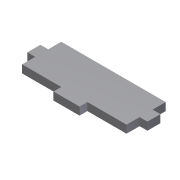
# Autodesk Inventor part: OpenROV_Dev_EChassis_Seperator
Saved by Autodesk Inventor 2012 (Build 160160000, 160)
## iProperties
Created: 2012-08-08
Part Number: OpenROV_Dev_EChassis_Seperator
Material: Default
Document SubType Name: Modeling
Designer: user
Density: 1 g/cm^3
Author: user
Autodesk Inventor part; units mm, degrees
ref_plane "YZ Plane" through (0, 0, 0) normal (1, 0, 0) x (0, 1, 0)
ref_plane "XZ Plane" through (0, 0, 0) normal (0, 1, 0) x (-1, 0, 0)
ref_plane "XY Plane" through (0, 0, 0) normal (0, 0, 1) x (1, 0, 0)
sketch "Sketch1" plane through (0, 0, 0) normal (0, 0, 1) x (1, 0, 0)
  line L0 (0, 0) -> (0, 5)
  line L1 (0, 5) -> (-3, 5)
  line L2 (-3, 5) -> (-3, 10)
  line L3 (0, 15) -> (40, 15)
  line L4 (43, 10) -> (43, 5)
  line L5 (43, 5) -> (40, 5)
  line L6 (40, 5) -> (40, 0)
  line L7 (40, 0) -> (25, 0)
  line L8 (25, 0) -> (25, -3)
  line L9 (25, -3) -> (15, -3)
  line L10 (15, -3) -> (15, 0)
  line L11 (15, 0) -> (0, 0)
  line L12 (40, 15) -> (40, 10)
  line L13 (40, 10) -> (43, 10)
  line L14 (-3, 10) -> (0, 10)
  line L15 (0, 10) -> (0, 15)
  dimension "d3" = 3
  dimension "d5" = 15
  dimension "d6" = 3
  dimension "d7" = 10
  dimension "d8" = 3
  dimension "d9" = 15
  dimension "d14" = 5
  dimension "d15" = 15
  dimension "d16" = 5
  dimension "d17" = 5
  dimension "d18" = 5
  dimension "d19" = 3
  dimension "d20" = 3
  constraints: 32 end point, 9 parallel, 4 perpendicular, 2 collinear, 1 vertical
  measures "d3" distance of L4.end L5.end
  measures "d5" distance of L6.end L7.end
  measures "d6" distance of L7.end L8.end
  measures "d7" distance of L8.end L9.end
  measures "d8" distance of L9.end L10.end
  measures "d9" distance of L10.end L0.start
  measures "d14" distance between parallel lines of L11 L1
  measures "d15" distance between parallel lines of L11 L3
  measures "d16" distance between parallel lines of L1 L14
  measures "d17" distance between parallel lines of L13 L5
  measures "d18" distance between parallel lines of L7 L5
  measures "d19" distance between parallel lines of L12 L4
  measures "d20" distance between parallel lines of L15 L2
extrude "Extrusion1" add sketch "Sketch1" along normal blind 3
body "Solid1"
